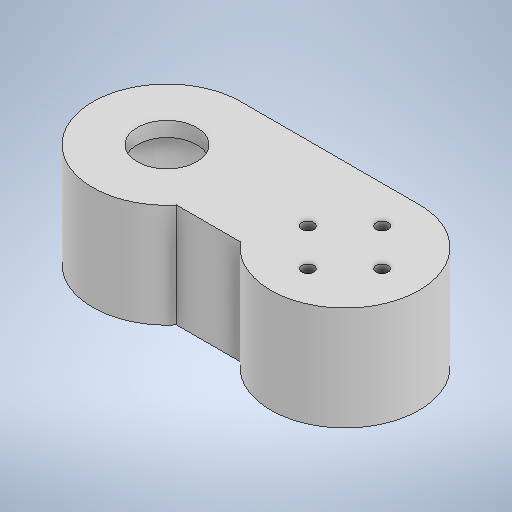
# Autodesk Inventor part: con_v7_d1
Saved by Autodesk Inventor 2025.4 (Build 294407000, 407)
## iProperties
Created: 2026-07-20
Part Number: con_v7_d1
Material: Generic
Document SubType Name: Modeling
Designer: Franchesca
Density: 1 g/cm^3
Appearance: Default
Author: Franchesca
## iProperties of the stored document con_v6_d1_3DPrint.ipt
Created: 2026-07-20
Part Number: con_v6_d1_3DPrint
Material: Generic
Document SubType Name: Modeling
Designer: Franchesca
Density: 1 g/cm^3
Appearance: Default
Author: Franchesca
Autodesk Inventor part; units mm, degrees
ref_plane "YZ Plane" through (0, 0, 0) normal (1, 0, 0) x (0, 1, 0)
ref_plane "XZ Plane" through (0, 0, 0) normal (0, 1, 0) x (-1, 0, 0)
ref_plane "XY Plane" through (0, 0, 0) normal (0, 0, 1) x (1, 0, 0)
sketch "Sketch1" plane through (0, 0, 0) normal (0, 1, 0) x (-1, 0, 0)
  line L0 (30, 0) -> (-30, 0) construction
  line L1 (30, 25) -> (-30, 25) construction
  line L2 (-30, -25) -> (30, -25)
  arc A0 (30, -25) -> (30, 25) centre (30, 0) ccw construction
  arc A1 (-30, 25) -> (-30, -25) centre (-30, 0) ccw
  line L3 (30, -25) -> (0, 0) construction
  line L4 (0, 0) -> (30, 25) construction
  line L5 (30, -25) -> (30, 25) construction
  line L6 (55, 0) -> (30, -25) construction
  line L7 (55, 0) -> (30, 25) construction
  line L8 (25, 25) -> (-25, 25) construction
  line L9 (-25, -25) -> (25, -25) construction
  arc A2 (25, -25) -> (25, 25) centre (25, 0) ccw construction
  line L10 (55, 0) -> (25, -25) construction
  line L11 (55, 0) -> (25, 25) construction
  line L12 (25, -25) -> (25, 25) construction
  line L13 (0, 0) -> (55, 0) construction
  circle A3 centre (-30, 0) radius 25 construction
  circle A4 centre (30, 0) radius 25 construction
  circle A5 centre (-30, 0) radius 22.5 construction
  line L14 (30, -25) -> (-30, -25)
  line L15 (0, -25) -> (0, 25) construction
  line L16 (30, 0) -> (0, 25) construction
  line L17 (10.7945, 16.0046) -> (-10.7945, 16.0046) construction
  line L18 (10.7945, 16.0046) -> (-10.7945, 16.0046)
  line L19 (8.9613, 13.5046) -> (-8.9613, 13.5046)
  circle A6 centre (30, 0) radius 10
  line L20 (19.1028, -22.5) -> (-19.1028, -22.5)
  circle A7 centre (-30, -12.5) radius 2
  circle A8 centre (-30, 12.5) radius 2
  line L21 (19.1028, -22.5) -> (19.0552, 22.4769) construction
  line L22 (10.7945, 16.0046) -> (10.7945, -22.5636) construction
  line L23 (10.7945, 16.0046) -> (49.3627, 16.0046) construction
  line L24 (-10.7945, 16.0046) -> (-10.7945, -22.0758) construction
  line L25 (-10.7945, 16.0046) -> (27.2859, 16.0046) construction
  line L26 (-10.7945, -22.0758) -> (-11.3044, -22.5) construction
  line L27 (-8.9613, 13.5046) -> (-8.9613, -22.5) construction
  line L28 (8.9613, 13.5046) -> (8.9613, -22.5) construction
  arc A9 (19.0998, -19.6834) -> (30, -22.5) centre (30, 0) ccw
  arc A10 (30, -22.5) -> (52.5, 0) centre (30, 0) ccw
  arc A11 (52.5, 0) -> (30, 22.5) centre (30, 0) ccw
  arc A12 (39.375, 20.4538) -> (19.0582, 19.6603) centre (30, 0) ccw
  circle A13 centre (30, 0) radius 22.5369 construction
  arc A14 (19.0582, 19.6603) -> (11.9574, 13.5046) centre (29.9457, -0.0723) ccw
  line L29 (8.9613, 13.5046) -> (11.9574, 13.5046)
  line L30 (19.0998, -19.6834) -> (19.1028, -22.5)
  arc A15 (30, 25) -> (10.7945, 16.0046) centre (30, 0) ccw
  arc A16 (55, 0) -> (30, 25) centre (30, 0) ccw
  arc A17 (30, -25) -> (55, 0) centre (30, 0) ccw
  arc A18 (-52.4985, -0.2589) -> (-19.1028, -19.685) centre (-30, 0) ccw
  arc A19 (-19.1028, 19.685) -> (-52.4985, -0.2589) centre (-30, 0) ccw
  line L31 (-8.9613, 13.5046) -> (-12.0035, 13.5046)
  arc A20 (-12.0035, 13.5046) -> (-19.1028, 19.685) centre (-30, 0) ccw
  line L32 (-19.1028, -22.5) -> (-19.1028, -19.685)
  arc A21 (-10.7945, 16.0046) -> (-30, 25) centre (-30, 0) ccw
  line L33 (-30, -12.5) -> (-30, 12.5) construction
  line L34 (-30, 0) -> (-42.5, 0) construction
  line L35 (-30, 0) -> (-17.5, 0) construction
  line L36 (-30, 0) -> (-17.5, 0) construction
  circle A22 centre (-17.5, 0) radius 2
  circle A23 centre (-42.5, 0) radius 2
  line L37 (-30, 0) -> (-30, -12.5) construction
  point P0 (-30, 25)
  point P1 (-25, 0)
  dimension "d1" = 30
  dimension "d2" = 50
  dimension "d3" = 50
  dimension "d9" = 50
  dimension "d12" = 45
  dimension "d13" = 0
  dimension "d14" = 2.5
  dimension "d15" = 20
  dimension "d16" = 2.5
  dimension "d25" = 4
  dimension "d28" = 4
  dimension "d29" = 90
  dimension "d30" = 90
  dimension "d51" = 25
  dimension "d53" = 12.5
  dimension "d60" = 12.5
  dimension "d61" = 180
  dimension "d62" = 12.5
  dimension "d63" = 4
  dimension "d64" = 4
  dimension "d65" = 12.5
  constraints: 78 end point, 50 point on circle, 23 centre point, 12 point on line, 8 coincident, 7 concentric, 7 horizontal, 7 tangent, 4 collinear, 4 midpoint, 3 equal length, 3 parallel, 3 perpendicular, 3 vertical, 4 other
  measures "d1" distance of L3.end L0.end
  measures "d2" diameter of A1
  measures "d3" distance between parallel lines of L1 L2
  measures "d9" diameter of A4
  measures "d12" diameter of A5
  measures "d13" distance between parallel lines of L9 L2
  measures "d14" distance between parallel lines of L17 L19
  measures "d15" diameter of A6
  measures "d16" distance between parallel lines of L20 L9
  measures "d25" diameter of A7
  measures "d28" diameter of A8
  measures "d29" angle of L22 L23
  measures "d30" angle of L24 L25
  measures "d51" distance of L33.end L33.start
  measures "d53" distance of A18.centre L33.start
  measures "d60" distance of L34.start L34.end
  measures "d61" angle of L34 L35
  measures "d62" distance of L34.start L35.end
  measures "d63" diameter of A22
  measures "d64" diameter of A23
  measures "d65" distance of L34.start L33.start
ref_plane "Work Plane1" through (0, -5, 0) normal (0, -1, 0) x (1, 0, 0)
extrude "Extrusion2" add sketch "Sketch1" against normal blind 35 contours A1 A21 L18 A15 A16 A17 L2
extrude "Extrusion3" add sketch "Sketch1" against normal blind 5 contours L29 A14 A12 A11 A10 A9 L30 L20 L32 A18 A19 A20 L31 L19 | A22 | A23
sketch "Sketch3" plane through (0, -35, 0) normal (0, -1, 0) x (1, 0, 0)
  point P0 (0, 0)
ref_plane "Work Plane2" through (0, -35, 0) normal (0, -1, 0) x (1, 0, 0)
sketch "Sketch4" plane through (0, -35, 0) normal (0, -1, 0) x (1, 0, 0)
  line L0 (0, 0) -> (-55, 0) construction
  arc A0 (-10.7945, 16.0046) -> (-30, -25) centre (-30, 0) ccw construction
  arc A1 (30, -25) -> (10.7945, 16.0046) centre (30, 0) ccw construction
  line L1 (0, 0) -> (55, 0) construction
  line L2 (-30, -25) -> (-30, 25) construction
  line L3 (30, -25) -> (30, 25) construction
  line L4 (-30, 13.5046) -> (30, 13.5046) construction
  line L5 (-19.1028, -22.5) -> (-19.0998, -19.6834) construction
  line L6 (-19.0998, -19.6834) -> (-30, -19.6834) construction
  arc A2 (-19.0582, 19.6603) -> (-19.0998, -19.6834) centre (-30, 0) ccw construction
  line L7 (-19.0998, -19.6834) -> (30, -19.6834) construction
  circle A3 centre (-53.8, 0) radius 0.75
  circle A4 centre (53.8, 0) radius 0.75
  arc A5 (19.1028, -19.685) -> (12.0035, 13.5046) centre (30, 0) ccw construction
  line L8 (-10.7945, 16.0046) -> (-10.7945, 13.5046) construction
  line L9 (10.7945, 16.0046) -> (10.7945, 13.5046) construction
  circle A6 centre (-10.7945, 14.7546) radius 0.75
  circle A7 centre (10.7945, 14.7546) radius 0.75
  point P0 (-52.5, 0.0238)
  point P1 (-52.5, 0.0238)
  dimension "d41" = 2.5
  dimension "d42" = 1.5
  dimension "d43" = 1.3
  dimension "d44" = 1.5
  dimension "d45" = 0.55
  dimension "d46" = 1.5
  dimension "d47" = 1.5
  dimension "d48" = 20.0889
  constraints: 18 end point, 9 point on line, 6 point on circle, 5 perpendicular, 4 centre point, 2 horizontal, 2 midpoint, 1 parallel
  measures "d41" horizontal distance of L0.end point (-52.5, 0.024)
  measures "d42" diameter of A3
  measures "d43" horizontal distance of A3.centre point (-52.5, 0.024)
  measures "d44" diameter of A4
  measures "d46" diameter of A6
  measures "d47" diameter of A7
extrude "Extrusion4" cut sketch "Sketch4" against normal blind 5
extrude "Extrusion5" cut sketch "Sketch1" against normal blind 5 contours A22 | A23
body "Solid2"
